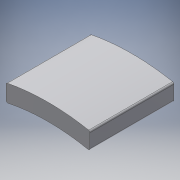
# Autodesk Inventor part: arc_magnet_10_10_2
Saved by Autodesk Inventor 2019.4 (Build 234330000, 330)
## iProperties
Created: 2019-10-01
Part Number: arc_magnet_10_10_2
Material: Generic
Document SubType Name: Modeling
Designer: cdi
Density: 1 g/cm^3
Appearance: White
Author: cdi
Autodesk Inventor part; units mm, degrees
ref_plane "YZ Plane" through (0, 0, 0) normal (1, 0, 0) x (0, 1, 0)
ref_plane "XZ Plane" through (0, 0, 0) normal (0, 1, 0) x (-1, 0, 0)
ref_plane "XY Plane" through (0, 0, 0) normal (0, 0, 1) x (1, 0, 0)
sketch "Sketch1" plane through (0, 0, 0) normal (0, 0, 1) x (1, 0, 0)
  arc A0 (5, 27.0925) -> (-5, 27.0925) centre (0, 0) ccw
  arc A1 (5, 25.056) -> (-5, 25.056) centre (0, 0) ccw
  line L0 (0, 0) -> (0, 34.5518)
  line L1 (-5, 0) -> (-5, 34.5518)
  line L2 (5, 0) -> (5, 34.5518)
  dimension "d0" = 55.1
  dimension "d1" = 2
  dimension "d2" = 10
  dimension "d3" = 5
  constraints: 6 end point, 4 point on circle, 4 point on line, 2 centre point, 2 coincident, 2 parallel, 1 vertical
  measures "d0" diameter of A0
  measures "d1" radial gap between concentric circles of A0 A1
  measures "d2" distance between parallel lines of L1 L2
  measures "d3" distance between parallel lines of L2 L0
extrude "Extrusion1" add sketch "Sketch1" along normal blind 10
fillet "Fillet1" radius 0.2 4 edges at (5, 27.0925, 5) (5, 25.056, 5) (-5, 27.0925, 5) (-5, 25.056, 5)
equation "\"d3\" = 0.5 * d2"
body "Solid1"
